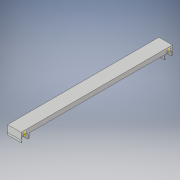
# Autodesk Inventor part: Horizontal Bar (9.25)
Saved by Autodesk Inventor 2018 (Build 220112000, 112)
## iProperties
Created: 2018-09-26
Part Number: Horizontal Bar (9.25)
Material: Generic
Document SubType Name: Modeling
Designer: Aditya Kendre
Density: 1 g/cm^3
Appearance: Default
Author: Aditya Kendre
Autodesk Inventor part; units mm, degrees
ref_plane "YZ Plane" through (0, 0, 0) normal (1, 0, 0) x (0, 1, 0)
ref_plane "XZ Plane" through (0, 0, 0) normal (0, 1, 0) x (-1, 0, 0)
ref_plane "XY Plane" through (0, 0, 0) normal (0, 0, 1) x (1, 0, 0)
sketch "Sketch1" plane through (0, 0, 0) normal (0, 1, 0) x (-1, 0, 0)
  line L0 (0, 0) -> (9.525, 0)
  line L1 (9.525, 0) -> (9.525, -101.6)
  line L2 (9.525, -101.6) -> (0, -101.6)
  line L3 (0, -101.6) -> (0, 0)
  dimension "d0" = 9.525
  dimension "d1" = 101.6
  constraints: 8 end point, 2 parallel, 1 horizontal, 1 perpendicular
  measures "d0" distance of L1.end L2.end
  measures "d1" distance of L0.end L1.end
extrude "Extrusion1" add sketch "Sketch1" along normal blind 3.175
sketch "Sketch2" plane through (0, 0, 0) normal (1, 0, 0) x (0, 0, -1)
  line L0 (0, 0) -> (0, 3.175) projected
  line L1 (101.6, 0) -> (101.6, 3.175) projected
  point P0 (0, 1.5875)
  point P1 (101.6, 1.5875)
  constraints: 2 midpoint
sketch "Sketch3" plane through (0, 0, -101.6) normal (0, 0, -1) x (-1, 0, 0)
  line L0 (9.525, 3.175) -> (0, 3.175) projected
  line L1 (0, 0) -> (9.525, 0) projected
  line L2 (9.525, 3.175) -> (0, 3.175)
  line L3 (0, 3.175) -> (0, 0)
  line L4 (0, 0) -> (9.525, 0)
  line L5 (9.525, 0) -> (9.525, 3.175)
  constraints: 8 end point, 2 parallel, 1 horizontal, 1 perpendicular
extrude "Extrusion2" add sketch "Sketch3" along normal blind 2.54
sketch "Sketch4" plane through (0, 0, 0) normal (0, -1, 0) x (1, 0, 0)
  point P0 (0, 0)
sketch "Sketch5" plane through (-9.525, 0, 0) normal (0, 0, 1) x (1, 0, 0)
  line L0 (0, 3.175) -> (9.525, 3.175) projected
  line L1 (0, 0) -> (9.525, 0)
  line L2 (9.525, 0) -> (9.525, 3.175)
  line L3 (9.525, 3.175) -> (0, 3.175)
  line L4 (0, 3.175) -> (0, 0)
  constraints: 8 end point, 2 parallel, 1 horizontal, 1 perpendicular
extrude "Extrusion3" add sketch "Sketch5" along normal blind 2.54
sketch "Sketch6" plane through (0, 0, 0) normal (0, -1, 0) x (1, 0, 0)
  line L0 (0, -104.14) -> (0, 2.54) projected
  line L1 (-9.525, 2.54) -> (-9.525, -104.14) projected
  line L2 (0, 2.54) -> (-9.525, 2.54)
  line L3 (-9.525, 2.54) -> (-9.525, -3.048)
  line L4 (-9.525, -3.048) -> (0, -3.048)
  line L5 (0, -3.048) -> (0, 2.54)
  line L6 (0, -104.14) -> (-9.525, -104.14)
  line L7 (-9.525, -104.14) -> (-9.525, -98.552)
  line L8 (-9.525, -98.552) -> (0, -98.552)
  line L9 (0, -98.552) -> (0, -104.14)
  point P0 (0, 0)
  dimension "d8" = 5.588
  dimension "d9" = 5.588
  constraints: 16 end point, 4 parallel, 2 horizontal, 2 perpendicular, 2 point on line
  measures "d8" distance of L3.end L2.end
  measures "d9" distance of L6.end L7.end
extrude "Extrusion4" add sketch "Sketch6" along normal blind 3.175 contours L6 L1 L8 L0 | L4 L1 L2 L0
sketch "Sketch7" plane through (-9.525, 3.175, -104.14) normal (-1, 0, 0) x (0, 0, 1)
  circle A0 centre (2.794, -4.7625) radius 2.54
  circle A1 centre (104.14, -4.7625) radius 2.54
  circle A2 centre (2.794, -4.7625) radius 2.54
  circle A3 centre (104.14, -4.7625) radius 2.54
  point P0 (104.14, -3.175)
  dimension "d12" = 5.08
  constraints: 4 centre point, 2 coincident, 2 concentric
  measures "d12" diameter of A0
hole "Hole1" at (-9.525, -1.5875, -101.346) at (-9.525, -1.5875, 0) direction (1, 0, 0) diameter 5.08 depth 25.4 tip angle 118
body "Solid1"
